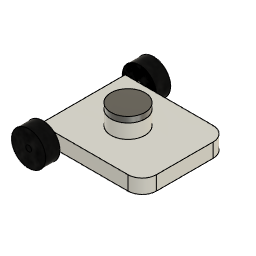
simplebot v8 (Autodesk Fusion 360 design; units mm, degrees)
Autodesk Fusion 360 part; units mm, degrees
sketch "Boceto1" plane through (0, 0, 0) normal (0, 0, 1) x (1, 0, 0)
  line L0 (-100, 75) -> (100, 75)
  line L1 (100, 75) -> (100, -75)
  line L2 (100, -75) -> (-100, -75)
  line L3 (-100, -75) -> (-100, 75)
  line L4 (-100, 75) -> (100, -75) construction
  line L5 (100, 75) -> (-100, -75) construction
  dimension "d1" = 200
  dimension "d2" = 150
  constraint horizontal L0
  constraint perpendicular L0 L1
  constraint parallel L0 L2
  constraint parallel L1 L3
  constraint coincident L4 origin
  constraint coincident L5 origin
  measures "d1" distance of L1.end L2.end
  measures "d2" distance of L0.end L1.end
extrude "Extrude1" add sketch "Boceto1" along normal blind 25 makes body 1
sketch "Sketch2" plane through (0, -75, 0) normal (0, -1, 0) x (1, 0, 0)
  line L0 (-100, 0) -> (100, 0)
  line L1 (100, 0) -> (100, 25)
  line L2 (100, 25) -> (-100, 25)
  line L3 (-100, 25) -> (-100, 0)
  line L4 (-100, 12.5) -> (-65, 12.5)
  circle A0 centre (-65, 12.5) radius 5
  dimension "d5" = 10
  constraint midpoint L3 L4.start
  constraint perpendicular L3 L4
  constraint coincident L4.end A0.centre
  measures "d5" diameter of A0
extrude "Extrude2" add sketch "Sketch2" along normal blind 10 contours A0 bodies 1
sketch "Sketch3" plane through (0, -85, 0) normal (0, -1, 0) x (1, 0, 0)
  circle A0 centre (-65, 12.5) radius 5
  circle A1 centre (-65, 12.5) radius 30
  dimension "d8" = 60
  constraint concentric A0 A1
  measures "d8" diameter of A1
extrude "Extrude3" add sketch "Sketch3" along normal blind 25 separate body makes body 2
mirror "Mirror1" about plane through (0, 0, 0) normal (0, 1, 0) of "Extrude2", "Extrude3" makes body 3
move_body "Move1" bodies 3 2 1 to x (1, 0, 0) y (0, 1, 0) z (0, 0, 1) at (0, 0, 17.5)
sketch "Sketch4" plane through (0, 0, 17.5) normal (0, 0, -1) x (1, 0, 0)
  line L0 (100, 75) -> (-100, 75)
  line L1 (-100, 75) -> (-100, -75)
  line L2 (-100, -75) -> (100, -75)
  line L3 (100, -75) -> (100, 75)
  line L4 (100, 0) -> (70, 0)
  circle A0 centre (70, 0) radius 15
  dimension "d14" = 30
  dimension "d15" = 30
  constraint midpoint L3 L4.start
  constraint perpendicular L3 L4
  constraint coincident L4.end A0.centre
  measures "d14" distance of L4.start L4.end
  measures "d15" diameter of A0
extrude "Extrude4" add sketch "Sketch4" along normal blind 17.5 separate body contours A0 makes body 4
fillet "Fillet1" radius 15 1 faces at (69.464, -3.9092, 0) on bodies 4
sketch "Sketch5" plane through (0, 0, 42.5) normal (0, 0, 1) x (-1, 0, 0)
  line L0 (100, 75) -> (-100, 75)
  line L1 (-100, 75) -> (-100, -75)
  line L2 (-100, -75) -> (100, -75)
  line L3 (100, -75) -> (100, 75)
  circle A0 centre (0, 0) radius 30
  dimension "d20" = 60
  constraint coincident A0.centre origin
  measures "d20" diameter of A0
extrude "Extrude5" add sketch "Sketch5" along normal blind 25 contours A0 bodies 1
extrude "Extrude6" add 1 faces at (-7.6631, -11.2397, 67.5) along direction (0, 0, 1) blind 10 separate body on bodies 1 makes body 5
chamfer "Chamfer1" distance 20 angle 45 1 edges at (-100, 0, 42.5) on bodies 1
fillet "Fillet2" radius 25 1 edges at (100, -75, 30) on bodies 1
fillet "Fillet3" radius 25 1 edges at (100, 75, 30) on bodies 1
copy_body "Body->Comp1" bodies 1 removing the originals makes body 6 in component "old_component"
copy_body "Body->Comp2" bodies 2 removing the originals makes body 7 in component "old_component (1)"
copy_body "Body->Comp3" bodies 3 removing the originals makes body 8 in component "old_component (2)"
copy_body "Body->Comp4" bodies 4 removing the originals makes body 9 in component "old_component (3)"
copy_body "Body->Comp5" bodies 5 removing the originals makes body 10 in component "old_component (4)"
move_body "Move1'" bodies 8 to x (1, 0, 0) y (0, 1, 0) z (0, 0, 1) at (0, 23, 0) in component "old_component (2)"
move_body "Move1''" bodies 10 to x (1, 0, 0) y (0, 1, 0) z (0, 0, 1) at (0, 0, 50) in component "old_component (4)"
copy_body "CopyPasteBodies1" bodies 6 makes body 11 in component "base_link"
copy_body "CopyPasteBodies1'" bodies 7 makes body 12 in component "right_wheel_1"
copy_body "CopyPasteBodies1''" bodies 8 body 8 seen with x (1, 0, 0) y (0, 1, 0) z (0, 0, 1) at (0, -23, 0) makes body 13 in component "left_wheel_1"
copy_body "CopyPasteBodies1'''" bodies 9 body 9 seen with x (-0.258819, -0.965926, 0) y (0.965926, -0.258819, 0) z (0, 0, 1) at (88.1173, 67.6148, 0) makes body 14 in component "caster_wheel_1"
copy_body "CopyPasteBodies1''''" bodies 10 body 10 seen with x (1, 0, 0) y (0, 1, 0) z (0, 0, 1) at (0, 0, -50) makes body 15 in component "lidar_1"
component "old_component" placed x (1, 0, 0) y (0, 1, 0) z (0, 0, 1) at (0, 0, 0)
component "old_component (1)" placed x (1, 0, 0) y (0, 1, 0) z (0, 0, 1) at (0, 0, 0)
component "old_component (2)" placed x (1, 0, 0) y (0, 1, 0) z (0, 0, 1) at (0, -23, 0)
component "old_component (3)" placed x (-0.258819, -0.965926, 0) y (0.965926, -0.258819, 0) z (0, 0, 1) at (88.1173, 67.6148, 0)
component "old_component (4)" placed x (1, 0, 0) y (0, 1, 0) z (0, 0, 1) at (0, 0, -50)
component "base_link" placed x (1, 0, 0) y (0, 1, 0) z (0, 0, 1) at (0, 0, 0)
component "right_wheel_1" placed x (1, 0, 0) y (0, 1, 0) z (0, 0, 1) at (0, 0, 0)
component "left_wheel_1" placed x (1, 0, 0) y (0, 1, 0) z (0, 0, 1) at (0, 0, 0)
component "caster_wheel_1" placed x (1, 0, 0) y (0, 1, 0) z (0, 0, 1) at (0, 0, 0)
component "lidar_1" placed x (1, 0, 0) y (0, 1, 0) z (0, 0, 1) at (0, 0, 0)
named bodies: "base_link", "left_wheel", "right_wheel", "caster_wheel", "lidar"
